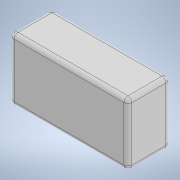
# Autodesk Inventor part: Battery Pack
Saved by Autodesk Inventor 2022.2 (Build 262287030, 287C)
## iProperties
Created: 2022-03-03
Part Number: Battery Pack
Material: Generic
Document SubType Name: Modeling
Designer: Jochen
Density: 1 g/cm^3
Appearance: Default
Author: Jochen
Autodesk Inventor part; units mm, degrees
ref_plane "YZ Plane" through (0, 0, 0) normal (1, 0, 0) x (0, 1, 0)
ref_plane "XZ Plane" through (0, 0, 0) normal (0, 1, 0) x (-1, 0, 0)
ref_plane "XY Plane" through (0, 0, 0) normal (0, 0, 1) x (1, 0, 0)
sketch "Sketch1" plane through (0, 0, 0) normal (0, 0, 1) x (1, 0, 0)
  line L0 (0, -21.7) -> (0, 21.7) construction
  line L1 (-41.3, 0) -> (41.3, 0) construction
  line L2 (-29.5, -15.5) -> (29.5, -15.5)
  line L3 (29.5, -15.5) -> (29.5, 15.5)
  line L4 (29.5, 15.5) -> (-29.5, 15.5)
  line L5 (-29.5, 15.5) -> (-29.5, -15.5)
  line L6 (-29.5, -15.5) -> (29.5, 15.5) construction
  line L7 (29.5, -15.5) -> (-29.5, 15.5) construction
  point P0 (0, 0)
  dimension "d0" = 59
  dimension "d1" = 31
  constraints: 12 end point, 2 midpoint, 2 parallel, 1 horizontal, 1 perpendicular
  measures "d0" distance of L4.end L3.end
  measures "d1" distance of L4.end L2.start
extrude "Extrusion1" add sketch "Sketch1" along normal blind 21
fillet "Fillet1" radius 2 12 edges at (0, 15.5, 21) (0, 15.5, 0) (29.5, 15.5, 10.5) (29.5, 0, 21) (29.5, 0, 0) (29.5, -15.5, 10.5) (0, -15.5, 21) (-29.5, 0, 21) (-29.5, -15.5, 10.5) (-29.5, 0, 0) (0, -15.5, 0) (-29.5, 15.5, 10.5)
body "Solid1"
